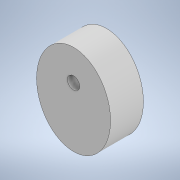
# Autodesk Inventor part: OVAAAAAL cam
Saved by Autodesk Inventor 2021 (Build 250183000, 183)
## iProperties
Created: 2021-04-14
Part Number: OVAAAAAL cam
Material: Generic
Document SubType Name: Modeling
Designer: Nabeel Azafer
Density: 1 g/cm^3
Appearance: Default
Author: Nabeel Azafer
Autodesk Inventor part; units mm, degrees
ref_plane "YZ Plane" through (0, 0, 0) normal (1, 0, 0) x (0, 1, 0)
ref_plane "XZ Plane" through (0, 0, 0) normal (0, 1, 0) x (-1, 0, 0)
ref_plane "XY Plane" through (0, 0, 0) normal (0, 0, 1) x (1, 0, 0)
sketch "Sketch1" plane through (0, 0, 0) normal (0, 0, 1) x (1, 0, 0)
  ellipse E0 centre (0, 0) end of major axis (0, 11) minor radius 9
  circle A0 centre (0, 3.5) radius 1.5
  dimension "d0" = 9
  dimension "d1" = 11
  dimension "d2" = 3
  dimension "d3" = 3.5
  constraints: 1 centre point, 1 coincident, 2 other
  measures "d2" diameter of A0
  measures "d3" distance of point (0, 0) A0.centre
extrude "Extrusion1" add sketch "Sketch1" along normal blind 8
body "Solid1"
